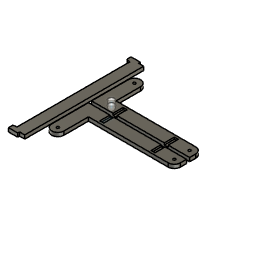
convertible_shelf (Autodesk Fusion 360 design; units mm, degrees)
Autodesk Fusion 360 part; units mm, degrees
sketch "Sketch1" plane through (0, 0, 0) normal (0, 0, 1) x (1, 0, 0)
  line L0 (0, 0) -> (12.5608, 0)
  spline S0 degree 3 poles (12.5608, 0) (14.7663, 0) (14.8331, -1.9054) (15.0336, -2.9747) knots 0 0 0 0 1 1 1 1
  spline S1 degree 2 poles (15.0336, -2.9747) (15.2341, -4.0441) (16.1249, -12) knots 0 0 0 1 1 1
  line L1 (16.1249, -12) -> (383.874, -12)
  spline S2 degree 2 poles (383.874, -12) (384.765, -4.0441) (384.965, -2.9747) knots 0 0 0 1 1 1
  spline S3 degree 3 poles (384.965, -2.9747) (385.166, -1.9054) (385.233, 0) (387.438, 0) knots 0 0 0 0 1 1 1 1
  line L2 (387.438, 0) -> (399.999, 0)
  line L3 (399.999, 0) -> (399.999, -29.9999)
  line L4 (399.999, -29.9999) -> (393.999, -29.9999)
  line L5 (393.999, -29.9999) -> (393.999, -46.9999)
  line L6 (393.999, -46.9999) -> (6, -46.9999)
  line L7 (6, -46.9999) -> (6, -29.9999)
  line L8 (6, -29.9999) -> (0, -29.9999)
  line L9 (0, -29.9999) -> (0, 0)
sketch "Sketch2" plane through (0, 0, 0) normal (0, 0, 1) x (1, 0, 0)
  line L0 (0, 0) -> (320, 0)
  line L1 (320, 0) -> (320, -20)
  line L2 (300, -40) -> (0, -40)
  line L3 (0, -40) -> (0, 0)
  line L4 (0, 0) -> (40, 0)
  line L5 (40, 0) -> (40, -120)
  line L6 (0, -120) -> (0, 0)
  circle A0 centre (20, -120) radius 4.15
  circle A1 centre (300, -20) radius 4.15
  arc A2 (0, -120) -> (20, -140) centre (20, -120) ccw
  arc A3 (20, -140) -> (40, -120) centre (20, -120) ccw
  arc A4 (300, -40) -> (320, -20) centre (300, -20) ccw
  point P0 (0, -140)
  dimension "d1" = 320
  dimension "d2" = 40
  dimension "d3" = 140
  dimension "d4" = 8.3
  dimension "d5" = 8.3
  dimension "d6" = 20
  dimension "d7" = 20
  constraint horizontal L0
  constraint vertical L1
  constraint horizontal L2
  constraint vertical L3
  constraint coincident L0.start L3.end
  constraint horizontal L4
  constraint vertical L5
  constraint vertical L6
  constraint coincident P0 L6
  constraint tangent L6 A2
  constraint tangent L5 A3
  constraint equal A2 A3
  constraint coincident A2.end A3.start
  constraint tangent L1 A4
  constraint tangent L2 A4
  measures "d1" distance of L0.start L0.end
  measures "d2" distance of L0.start L4.end
  measures "d3" distance of L0.start P0
  measures "d4" diameter of A0
  measures "d5" diameter of A1
  measures "d6" radius of A2
  measures "d7" radius of A4
extrude "Extrude1" add sketch "Sketch2" along normal blind 12 makes body 1
move_body "Move1" bodies 1 to x (1, 0, 0) y (0, 1, 0) z (0, 0, 1) at (-45, 45, 0)
extrude "Extrude2" add sketch "Sketch1" along normal blind 12 separate body makes body 2
sketch "Sketch3" plane through (0, 0, 12) normal (0, 0, 1) x (-1, 0, 0)
  circle A0 centre (-255, -25) radius 4.15
  circle A1 centre (25, 75) radius 4.15
  line L0 (5, -5) -> (-255, -5)
  arc A2 (-255, -5) -> (-275, -25) centre (-255, -25) ccw
  line L1 (-275, -25) -> (-275, -45)
  line L2 (-275, -45) -> (45, -45)
  line L3 (45, -45) -> (45, 75)
  arc A3 (45, 75) -> (5, 75) centre (25, 75) ccw
  line L4 (5, 75) -> (5, -5)
  line L5 (45, -45) -> (-25, -45)
  line L6 (-25, -45) -> (-25, -60)
  line L7 (-25, -60) -> (45, -60)
  line L8 (45, -60) -> (45, -45)
  line L9 (-275, -45) -> (-205, -45)
  line L10 (-205, -45) -> (-205, -61)
  line L11 (-205, -61) -> (-275, -61)
  line L12 (-275, -61) -> (-275, -45)
  line L13 (-25, -45) -> (-37.7, -45)
  line L14 (-37.7, -45) -> (-37.7, -12)
  line L15 (-37.7, -12) -> (-25, -12)
  line L16 (-25, -12) -> (-25, -45)
  line L17 (-205, -45) -> (-192.3, -45)
  line L18 (-192.3, -45) -> (-192.3, -12)
  line L19 (-192.3, -12) -> (-205, -12)
  line L20 (-205, -12) -> (-205, -45)
  dimension "d15" = 70
  dimension "d16" = 70
  dimension "d17" = 12.7
  dimension "d18" = 33
  dimension "d19" = 12.7
  dimension "d20" = 33
  constraint horizontal L5
  constraint vertical L6
  constraint horizontal L7
  constraint vertical L8
  constraint coincident L2.end L3.start
  constraint horizontal L9
  constraint vertical L10
  constraint horizontal L11
  constraint vertical L12
  constraint coincident L1.end L2.start
  constraint horizontal L13
  constraint vertical L14
  constraint horizontal L15
  constraint vertical L16
  constraint horizontal L17
  constraint vertical L18
  constraint horizontal L19
  constraint vertical L20
  measures "d15" distance of L2.end L5.end
  measures "d16" distance of L1.end L9.end
  measures "d17" distance of L5.end L13.end
  measures "d18" distance of L5.end L15.end
  measures "d19" distance of L9.end L17.end
  measures "d20" distance of L9.end L19.end
extrude "Extrude3" cut sketch "Sketch3" against normal blind 6 contours L2 L17 L18 L19 L20 | L2 L13 L14 L15 L16 bodies 1
sketch "Sketch4" plane through (0, 0, 6) normal (0, 0, 1) x (-1, 0, 0)
  line L0 (-25, -12) -> (-37.7, -12)
  line L1 (-37.7, -12) -> (-37.7, -45)
  line L2 (-37.7, -45) -> (-25, -45)
  line L3 (-25, -45) -> (-25, -12)
  line L4 (0, -75) -> (15, -90)
move_body "Move3" bodies 2 to x (0, 1, 0) y (-1, 0, 0) z (0, 0, 1) at (346.9991, -440.9989, 0)
move_body "Move4" bodies 2 to x (1, 0, 0) y (0, 1, 0) z (0, 0, 1) at (-130, 210, 0)
sketch "Sketch5" plane through (0, 0, 0) normal (0, 0, 1) x (1, 0, 0)
mirror "Spiegeln1" about plane through (0, 0, 0) normal (0, 1, 0) of bodies 1 makes body 3
move_body "Verschieben5" bodies 3 to x (1, 0, 0) y (0, 1, 0) z (0, 0, 1) at (0, 100, 0)
move_body "Verschieben6" bodies 2 to x (1, 0, 0) y (0, 1, 0) z (0, 0, 1) at (-321.8977, 74.9046, 0)
